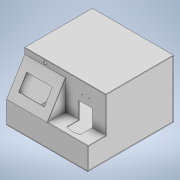
# Autodesk Inventor part: Vỏ
Saved by Autodesk Inventor 2020 (Build 240168000, 168)
## iProperties
Created: 2022-09-23
Part Number: Vỏ
Material: Generic
Document SubType Name: Modeling
Designer: ASUS
Density: 1 g/cm^3
Appearance: Default
Author: ASUS
Autodesk Inventor part; units mm, degrees
ref_plane "YZ Plane" through (0, 0, 0) normal (1, 0, 0) x (0, 1, 0)
ref_plane "XZ Plane" through (0, 0, 0) normal (0, 1, 0) x (-1, 0, 0)
ref_plane "XY Plane" through (0, 0, 0) normal (0, 0, 1) x (1, 0, 0)
sketch "Sketch7" plane through (0, 0, 0) normal (0, 0, 1) x (1, 0, 0)
  line L0 (0, 0) -> (600, 0)
  line L1 (600, 0) -> (600, 160)
  line L2 (600, 160) -> (0, 160)
  line L3 (0, 160) -> (0, 0)
  dimension "d13" = 600
  dimension "d14" = 160
  constraints: 8 end point, 2 parallel, 1 horizontal, 1 perpendicular
  measures "d13" distance of L2.end L1.end
  measures "d14" distance of L1.end L0.end
extrude "Extrusion4" add sketch "Sketch7" against normal blind 5
sketch "Sketch8" plane through (0, 0, -5) normal (0, 0, -1) x (-1, 0, 0)
  line L0 (-600, 160) -> (-600, 0) projected
  line L1 (-600, 160) -> (-300, 160)
  line L2 (-300, 160) -> (-300, 155)
  line L3 (-300, 155) -> (-600, 155)
  line L4 (-600, 155) -> (-600, 160)
  point P0 (0, 0)
  dimension "d17" = 300
  dimension "d18" = 5
  constraints: 8 end point, 2 parallel, 1 horizontal, 1 perpendicular
  measures "d17" distance of L2.end L3.end
  measures "d18" distance of L1.end L2.end
extrude "Extrusion5" add sketch "Sketch8" along normal blind 130
ref_plane "Work Plane1" through (0, 0, -5) normal (0, 0, -1) x (-1, 0, 0)
split body "Split1" result two bodies by plane through (0, 0, -5) normal (0, 0, -1) first body at (500, 159.5, -48.3333)
sketch "Sketch9" plane through (300, 160, -135) normal (0, 1, 0) x (1, 0, 0)
  line L0 (0, 0) -> (300, 0) projected
  line L1 (100, 0) -> (200, 0)
  arc A0 (100, -86.6025) -> (200, -86.6025) centre (150, 0) ccw
  line L2 (200, 0) -> (200, -86.6025)
  line L3 (100, -86.6025) -> (100, 0)
  point P0 (-300, -135)
  constraints: 6 end point, 2 point on circle, 1 centre point, 1 coincident, 1 midpoint, 1 parallel
extrude "Extrusion6" cut sketch "Sketch9" against normal through all bodies 2
sketch "Sketch10" plane through (0, 0, -135) normal (0, 0, -1) x (-1, 0, 0)
  line L0 (-300, 155) -> (-300, 420)
  line L1 (-300, 420) -> (-600, 420)
  line L2 (-600, 420) -> (-600, 155)
  line L3 (-400, 155) -> (-500, 155) projected
  line L4 (-500, 155) -> (-400, 155)
  line L5 (-400, 155) -> (-400, 285)
  line L6 (-400, 285) -> (-500, 285)
  line L7 (-500, 285) -> (-500, 155)
  line L8 (-600, 155) -> (-500, 155)
  line L9 (-400, 155) -> (-300, 155)
  line L10 (-450, 285) -> (-475, 285)
  circle A0 centre (-500, 285) radius 3
  circle A1 centre (-400, 285) radius 3
  point P0 (0, 0)
  dimension "d82" = 300
  dimension "d83" = 265
  dimension "d84" = 100
  dimension "d85" = 130
  constraints: 20 end point, 5 parallel, 4 horizontal, 3 perpendicular, 2 centre point, 1 midpoint
  measures "d82" distance of L1.end L0.end
  measures "d83" distance of L0.end L0.start
  measures "d84" distance of L6.end L5.end
  measures "d85" distance of L5.end L4.end
extrude "Extrusion7" add sketch "Sketch10" along normal blind 5 contours L9 L5 A1 L6 A0 L7 L8 L2 L1 L0 | L5 L6 A1 | A0 L6 L7 picked at (-400.9227, 286.758) picked at (-498.7173, 286.5144) bodies 2
ref_plane "Work Plane2" through (0, 0, -135) normal (0, 0, 1) x (1, 0, 0)
sketch "Sketch11" plane through (300, 155, -135) normal (-1, 0, 0) x (0, 0, 1)
  line L0 (-5, 265) -> (-5, 0) projected
  line L1 (-5, 265) -> (0, 265)
  line L2 (0, 265) -> (0, 225)
  line L3 (0, 225) -> (-5, 225)
  line L4 (-5, 225) -> (-5, 265)
  point P0 (135, -155)
  point P1 (-5, 225)
  dimension "d93" = 5
  dimension "d94" = 40
  constraints: 8 end point, 2 parallel, 1 horizontal, 1 perpendicular
  measures "d93" distance of L2.end L3.end
  measures "d94" distance of L1.end L2.end
extrude "Extrusion8" add sketch "Sketch11" along normal blind 300 separate body
sketch "Sketch12" plane through (0, 0, -135) normal (0, 0, 1) x (1, 0, 0)
  line L0 (0, 380) -> (0, 420) projected
  line L1 (300, 380) -> (0, 380) projected
  line L2 (0, 420) -> (300, 380)
  circle A0 centre (150, 400) radius 11.5
  circle A1 centre (475, 334.9293) radius 3
  circle A2 centre (425, 334.9293) radius 3
  line L3 (400, 285) -> (500, 285)
  line L4 (500, 285) -> (500, 335)
  line L5 (500, 335) -> (400, 335)
  line L6 (400, 335) -> (400, 285)
  point P0 (0, 0)
  dimension "d95" = 23
  dimension "d136" = 50
  constraints: 10 end point, 3 centre point, 2 parallel, 1 horizontal, 1 midpoint, 1 perpendicular
  measures "d95" diameter of A0
  measures "d136" distance of L4.end L3.end
extrude "Extrusion9" cut sketch "Sketch12" against normal blind 138.35 contours A0 L2 | L2 A0 | A1 L5 | L5 A1 | L5 A2 | A2 L5 bodies 4 2
sketch "Sketch13" plane through (0, 0, -5) normal (0, 0, -1) x (-1, 0, 0)
  line L0 (-600, 0) -> (-600, 160) projected
  line L1 (-300, 155) -> (-600, 155) projected
  line L2 (-600, 0) -> (-595, 0)
  line L3 (-595, 0) -> (-595, 155)
  line L4 (-595, 155) -> (-600, 155)
  line L5 (-600, 155) -> (-600, 0)
  line L6 (0, 160) -> (-5, 160)
  line L7 (-5, 160) -> (-5, 0)
  line L8 (-5, 0) -> (0, 0)
  line L9 (0, 0) -> (0, 160)
  dimension "d100" = 5
  dimension "d101" = 5
  dimension "d102" = 160
  constraints: 16 end point, 4 parallel, 2 horizontal, 2 perpendicular, 1 point on line
  measures "d100" distance of L4.end L3.end
  measures "d101" distance of L8.end L7.end
  measures "d102" distance of L7.end L6.end
extrude "Extrusion10" add sketch "Sketch13" along normal blind 630 bodies 3
ref_plane "Work Plane3" through (0, 0, -5) normal (0, 0, -1) x (-1, 0, 0)
ref_plane "Work Plane17" through (0, 0, -5) normal (0, 0, 1) x (1, 0, 0)
split body "Split19" result two bodies by plane through (0, 0, -5) normal (0, 0, 1) bodies 3 first body at (400, 53.3333, -0.5)
sketch "Sketch25" plane through (600, 155, -5) normal (0, 1, 0) x (1, 0, 0)
  line L0 (0, 0) -> (0, 630) projected
  line L1 (-5, 0) -> (-5, 630) projected
  line L2 (0, 630) -> (-5, 630)
  line L3 (-5, 630) -> (-5, 135)
  line L4 (-5, 135) -> (0, 135)
  line L5 (0, 135) -> (0, 630)
  point P0 (-600, -5)
  point P1 (0, 135)
  dimension "d105" = 495
  constraints: 8 end point, 2 parallel, 1 horizontal, 1 perpendicular, 1 point on line
  measures "d105" distance of L3.end L2.end
extrude "Extrusion19" add sketch "Sketch25" along normal blind 265 bodies 6
ref_plane "Work Plane18" through (5, 0, -635) normal (1, 0, 0) x (0, 0, -1)
split body "Split20" result two bodies by plane through (5, 0, -635) normal (1, 0, 0) bodies 6 first body at (599.5, 191.6667, -470)
ref_plane "Work Plane19" through (0, 0, -135) normal (0, 0, 1) x (1, 0, 0)
split body "Split21" result two bodies by plane through (0, 0, -135) normal (0, 0, 1) bodies 2 first body at (333.3333, 159.5, -62.7992)
sketch "Sketch26" plane through (0, 0, -635) normal (-1, 0, 0) x (0, 0, 1)
  line L0 (0, 0) -> (0, 420) projected
  line L1 (495, 420) -> (495, 380) projected
  line L2 (0, 420) -> (495, 420)
  line L3 (495, 380) -> (500, 380) projected
  line L4 (495, 420) -> (495, 380)
  line L5 (630, 0) -> (630, 160) projected
  line L6 (495, 380) -> (630, 160)
  line L7 (630, 160) -> (0, 160)
  line L8 (0, 160) -> (0, 420)
  point P0 (635, 0)
  constraints: 10 end point, 3 perpendicular, 1 parallel
extrude "Extrusion20" add sketch "Sketch26" against normal blind 5 bodies 8
sketch "Sketch27" plane through (0, 0, -635) normal (-1, 0, 0) x (0, 0, 1)
  line L0 (495, 380) -> (500, 380) projected
  line L1 (635, 160) -> (635, 0) projected
  line L2 (500, 380) -> (635, 160)
  line L3 (630, 160) -> (500, 160) projected
  line L4 (635, 160) -> (630, 160)
  line L5 (495, 380) -> (630, 160) projected
  line L6 (630, 160) -> (495, 380)
  line L7 (495, 380) -> (500, 380)
  constraints: 8 end point, 2 collinear, 1 parallel
ref_plane "Work Plane20" through (0, 160, -5) normal (0, -0.5230162, -0.8523227) x (0, 0.8523227, -0.5230162)
extrude "Extrusion21" add sketch "Sketch27" against normal blind 300 bodies 8
split body "Split22" result two bodies by plane through (0, 160, -5) normal (0, -0.5230162, -0.8523227) bodies 8 first body at (0.5, 266.6667, -470)
ref_plane "Work Plane21" through (0, 380, -135) normal (0, 1, 0) x (1, 0, 0)
split body "Split23" result two bodies by plane through (0, 380, -135) normal (0, 1, 0) bodies 12 first body at (0.5, 406.6667, -148.1818)
combine bodies "Combine5" operation type add bodies to combine 13 11
sketch "Sketch28" plane through (0, 160, 0) normal (0, 0.5230162, 0.8523227) x (1, 0, 0)
  line L0 (54.5, 180.2294) -> (245.5, 180.2294)
  line L1 (245.5, 180.2294) -> (245.5, 65.2294)
  line L2 (245.5, 65.2294) -> (54.5, 65.2294)
  line L3 (54.5, 65.2294) -> (54.5, 180.2294)
  line L4 (54.5, 180.2294) -> (245.5, 65.2294) construction
  line L5 (245.5, 180.2294) -> (54.5, 65.2294) construction
  line L6 (300, 258.1182) -> (300, 0) projected
  line L7 (0, -133.7566) -> (0, 195.7437) projected
  point P0 (0, -136.3716)
  point P1 (150, 122.7294)
  dimension "d114" = 191
  dimension "d115" = 115
  dimension "d116" = 150
  constraints: 12 end point, 2 midpoint, 2 parallel, 1 horizontal, 1 perpendicular
  measures "d114" distance of L1.end L2.end
  measures "d115" distance of L0.end L1.end
  measures "d116" distance from line of L6 point (150, 122.729)
extrude "Extrusion22" cut sketch "Sketch28" against normal blind 300 bodies 14
ref_plane "Work Plane22" through (300, 380, -135) normal (-1, 0, 0) x (0, 1, 0)
combine bodies "Combine6" operation type add bodies to combine 4 10
sketch "Sketch29" plane through (0, 0, 0) normal (0, -1, 0) x (1, 0, 0)
  line L0 (600, 0) -> (600, -5) projected
  line L1 (0, 0) -> (600, 0)
  line L2 (600, 0) -> (600, -5)
  line L3 (600, -5) -> (0, -5)
  line L4 (0, -5) -> (0, 0)
  constraints: 8 end point, 2 parallel, 1 horizontal, 1 perpendicular
extrude "Extrusion23" add sketch "Sketch29" along normal blind 5 bodies 5
ref_plane "Work Plane23" through (595, 0, -5) normal (0, -1, 0) x (0, 0, -1)
sketch "Sketch30" plane through (0, 0, -5) normal (0, 0, -1) x (-1, 0, 0)
  line L0 (-600, -5) -> (-600, 160) projected
  line L1 (-600, -5) -> (0, -5)
  line L2 (0, -5) -> (0, 0)
  line L3 (0, 0) -> (-600, 0)
  line L4 (-600, 0) -> (-600, -5)
  constraints: 8 end point, 2 parallel, 1 horizontal, 1 perpendicular
extrude "Extrusion24" add sketch "Sketch30" along normal blind 630 bodies 5
split body "Split24" result two bodies by plane through (595, 0, -5) normal (0, -1, 0) bodies 5 first body at (400, -4.5, -423.3333)
sketch "Sketch31" plane through (0, 0, 0) normal (0, 1, 0) x (1, 0, 0)
  line L0 (595, 5) -> (595, 635) projected
  line L1 (5, 635) -> (5, 140) projected
  line L2 (595, 635) -> (5, 635)
  line L3 (5, 635) -> (5, 630)
  line L4 (5, 630) -> (595, 630)
  line L5 (595, 630) -> (595, 635)
  point P0 (0, 0)
  point P1 (5, 635)
  dimension "d123" = 5
  constraints: 8 end point, 2 parallel, 1 horizontal, 1 perpendicular, 1 point on line
  measures "d123" distance of L3.end L2.end
extrude "Extrusion25" add sketch "Sketch31" along normal blind 420 bodies 15
ref_plane "Work Plane24" through (0, 0, 0) normal (0, 1, 0) x (1, 0, 0)
split body "Split25" result two bodies by plane through (0, 0, 0) normal (0, 1, 0) bodies 15 first body at (201.6667, 140, -634.5)
ref_plane "Work Plane25" through (0, 420, -140) normal (0, 1, 0) x (1, 0, 0)
ref_plane "Work Plane26" through (0, 0, -630) normal (0, 0, -1) x (-1, 0, 0)
split body "Split27" result two bodies by plane through (0, 0, -630) normal (0, 0, -1) bodies 7 first body at (595.5, 140, -633.3333)
split body "Split28" result two bodies by plane through (0, 0, -630) normal (0, 0, -1) bodies 13 first body at (3.3333, 280, -630.5)
sketch "Sketch33" plane through (300, 155, -140) normal (-1, 0, 0) x (0, 0, 1)
  line L0 (0, 225) -> (5, 225) projected
  line L1 (0, 225) -> (0, 0)
  line L2 (0, 0) -> (135, 0)
  line L3 (140, 5) -> (135, 5) projected
  line L4 (135, 0) -> (135, 5)
  line L5 (135, 0) -> (135, 5)
  line L6 (135, 5) -> (0, 225)
  point P0 (140, -155)
  constraints: 10 end point, 2 perpendicular, 2 vertical
extrude "Extrusion27" add sketch "Sketch33" along normal blind 5 bodies 4
ref_plane "Work Plane27" through (300, 155, -140) normal (1, 0, 0) x (0, 0, -1)
split body "Split29" result two bodies by plane through (300, 155, -140) normal (1, 0, 0) bodies 4 first body at (566.6667, 286.6667, -135.5)
ref_plane "Work Plane31" through (300, 380, -135) normal (0, 1, 0) x (1, 0, 0)
split body "Split31" result two bodies by plane through (300, 380, -135) normal (0, 1, 0) bodies 24 first body at (46.1667, 400, -135.5)
combine bodies "Combine10" operation type add bodies to combine 25 23
sketch "Sketch34" plane through (600, 420, -5) normal (0, 1, 0) x (1, 0, 0)
  line L0 (-600, 130) -> (-300, 130) projected
  line L1 (0, 630) -> (-5, 630) projected
  line L2 (-600, 130) -> (0, 130)
  line L3 (0, 130) -> (0, 630)
  line L4 (0, 630) -> (-600, 630)
  line L5 (-600, 630) -> (-600, 130)
  point P0 (-600, -5)
  constraints: 8 end point, 2 parallel, 1 horizontal, 1 perpendicular
combine bodies "Combine11" operation type add bodies to combine 17 19 21
extrude "Extrusion28" add sketch "Sketch34" along normal blind 5 bodies 20
ref_plane "Work Plane32" through (600, 420, -5) normal (0, 1, 0) x (1, 0, 0)
split body "Split32" result two bodies by plane through (600, 420, -5) normal (0, 1, 0) bodies 20 first body at (200, 424.5, -301.6667)
body "Solid49"
body "Solid61"
body "Solid63"
body "Solid64"
